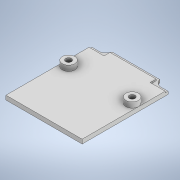
# Autodesk Inventor part: ExpansionCard_SelfTapping_Lid
Saved by Autodesk Inventor 2022 (Build 260153000, 153)
## iProperties
Created: 2022-05-23
Part Number: ExpansionCard_SelfTapping_Lid
Material: Generic
Document SubType Name: Modeling
Designer: SHOP-Station5
Density: 1 g/cm^3
Appearance: Default
Author: SHOP-Station5
Autodesk Inventor part; units mm, degrees
ref_plane "YZ Plane" through (0, 0, 0) normal (1, 0, 0) x (0, 1, 0)
ref_plane "XZ Plane" through (0, 0, 0) normal (0, 1, 0) x (-1, 0, 0)
ref_plane "XY Plane" through (0, 0, 0) normal (0, 0, 1) x (1, 0, 0)
sketch "Sketch1" plane through (0, 0, 0) normal (0, 1, 0) x (-1, 0, 0)
  line L0 (-27.0524, -30.5) -> (0, -30.5)
  line L1 (-27.0524, -30.5) -> (-27.0524, 0)
  line L2 (-27.0524, 0) -> (0, 0)
  line L3 (0, 0) -> (0, -30.5)
  point P0 (-13.5262, -30.5)
  constraints: 8 end point, 1 vertical
extrude "Extrusion1" add sketch "Sketch1" along normal blind 1.5
sketch "Sketch2" plane through (0, 0, 0) normal (0, -1, 0) x (1, 0, 0)
  circle A0 centre (2.2262, -20) radius 2.2262
  circle A1 centre (24.8262, -20) radius 2.2262
  point P0 (0, 0)
  point P1 (13.5262, -30.5)
  point P2 (27.0524, -30.5)
  constraints: 2 centre point
extrude "Extrusion2" add sketch "Sketch2" against normal blind 3.4
sketch "Sketch3" plane through (0, 0, 0) normal (0, -1, 0) x (1, 0, 0)
  circle A0 centre (24.8262, -19.9938) radius 1.016
  circle A1 centre (2.2262, -20) radius 1.016
  point P0 (0, 0)
  point P1 (13.5262, 0)
  point P2 (1.4262, -20)
  point P3 (0, -30.5)
  dimension "d4" = 2.032
  constraints: 2 centre point
  measures "d4" diameter of A0
extrude "Extrusion3" cut sketch "Sketch3" against normal up to surface (3.4 mm away)
sketch "Sketch4" plane through (0, 0, 0) normal (0, -1, 0) x (1, 0, 0)
  circle A0 centre (24.8262, -19.9938) radius 2.032
  circle A1 centre (2.2262, -20) radius 2.032
  line L0 (2.2262, -20) -> (0, -20)
  line L1 (0, -20) -> (0, -30.5)
  line L2 (0, -30.5) -> (0, 0) projected
  point P0 (13.5262, 0)
  dimension "d7" = 4.064
  dimension "d8" = 4.064
  constraints: 4 end point, 2 centre point, 1 coincident, 1 horizontal
  measures "d7" diameter of A0
  measures "d8" diameter of A1
extrude "Extrusion4" cut sketch "Sketch4" against normal blind 2.051
sketch "Sketch13" plane through (0, 1.5, 0) normal (0, 1, 0) x (1, 0, 0)
  arc A0 (22.0156, 32.63) -> (24.5977, 30.5) centre (24.5977, 33.13) ccw
  arc A1 (2.4547, 30.5) -> (5.0367, 32.63) centre (2.4547, 33.13) ccw
  line L0 (22.0156, 32.63) -> (5.0367, 32.63)
  arc A2 (2.4547, 30.5) -> (5.0367, 32.63) centre (2.4547, 33.13) ccw
  line L1 (27.0524, 20) -> (27.0524, 30.5) projected
  line L2 (2.4547, 30.5) -> (24.5977, 30.5)
  line L3 (27.0524, 30.5) -> (0, 30.5) projected
  point P0 (0, 0)
  point P1 (13.5262, 31)
  point P2 (24.5977, 30.5)
  constraints: 6 point on circle, 4 end point, 3 centre point, 1 coincident, 1 point on line
extrude "Extrusion11" add sketch "Sketch13" against normal up to surface (1.5 mm away)
sketch "Sketch14" plane through (0, 1.5, 0) normal (0, 1, 0) x (1, 0, 0)
  line L0 (27.0478, 29.5) -> (21.7177, 29.5)
  line L1 (21.7177, 31.63) -> (5.3347, 31.63)
  line L2 (21.7177, 31.63) -> (21.7177, 29.5)
  line L3 (21.7177, 31.63) -> (5.3347, 31.63)
  line L4 (5.3347, 31.63) -> (5.3347, 29.5)
  line L5 (0, 29.5) -> (4.5847, 29.5)
  line L6 (5.3347, 29.5) -> (4.5847, 29.5)
  line L7 (4.5847, 29.5) -> (0, 29.5)
  line L8 (2.4547, 30.5) -> (0, 30.5)
  line L9 (0, 29.5) -> (0, 30.5)
  line L10 (0, 30.5) -> (2.4547, 30.5)
  arc A0 (2.4547, 30.5) -> (5.0367, 32.63) centre (2.4547, 33.13) ccw
  line L11 (5.0367, 32.63) -> (22.0156, 32.63)
  line L12 (5.0367, 32.63) -> (22.0156, 32.63)
  line L13 (27.0524, 30.5) -> (27.0524, 29.5)
  line L14 (27.0524, 29.5) -> (27.0524, 30.5)
  line L15 (27.0524, 30.5) -> (24.5977, 30.5)
  arc A1 (22.0156, 32.63) -> (24.5977, 30.5) centre (24.5977, 33.13) ccw
  arc A2 (22.0156, 32.63) -> (24.5977, 30.5) centre (24.5977, 33.13) ccw
  arc A3 (2.4547, 30.5) -> (5.0367, 32.63) centre (2.4547, 33.13) ccw
  line L16 (27.0524, 30.5) -> (24.5977, 30.5) projected
  line L17 (0, 29.5) -> (5.3347, 29.5)
  line L18 (5.3347, 31.63) -> (5.3347, 29.5)
  line L19 (5.3347, 31.63) -> (21.7177, 31.63)
  line L20 (21.7177, 29.5) -> (21.7177, 31.63)
  line L21 (21.7177, 29.5) -> (27.0524, 29.5)
  line L22 (27.0524, 0) -> (27.0524, 30.5) projected
  line L23 (27.0524, 29.5) -> (27.0524, 30.5)
  arc A4 (22.0156, 32.63) -> (24.5977, 30.5) centre (24.5977, 33.13) ccw projected
  line L24 (27.0524, 30.5) -> (24.5977, 30.5)
  line L25 (22.0156, 32.63) -> (5.0367, 32.63) projected
  line L26 (22.0156, 32.63) -> (5.0367, 32.63)
  line L27 (2.4547, 30.5) -> (0, 30.5) projected
  line L28 (2.4547, 30.5) -> (0, 30.5)
  line L29 (0, 30.5) -> (0, 29.5)
  arc A5 (2.4547, 30.5) -> (5.0367, 32.63) centre (2.4547, 33.13) ccw
  arc A6 (22.0156, 32.63) -> (24.5977, 30.5) centre (24.5977, 33.13) ccw
  point P0 (0, 0)
  point P1 (13.5262, 31)
  constraints: 53 end point, 13 point on circle, 9 collinear, 8 perpendicular, 6 centre point, 4 coincident, 3 tangent, 1 concentric, 1 point on line
extrude "Extrusion12" cut sketch "Sketch14" against normal blind 0.5
body "Solid1"
